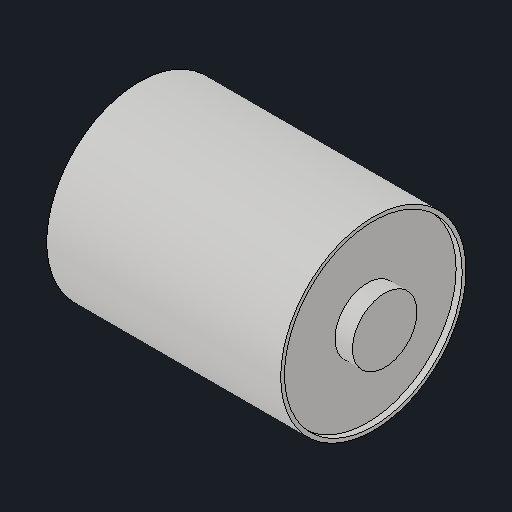
# Autodesk Inventor part: Silnik
Saved by Autodesk Inventor 2023 (Build 270158000, 158)
## iProperties
Created: 2022-01-30
Part Number: Silnik
Material: Ogólny
Document SubType Name: Modeling
Designer: Michał
Density: 4.22271 g/cm^3
Appearance: Domyślna
Mass: 60 g
Surface Area: 34.9646 cm^2
Volume: 14.2089 cm^3
Author: Michał
Autodesk Inventor part; units mm, degrees
ref_plane "YZ Plane" through (0, 0, 0) normal (1, 0, 0) x (0, 1, 0)
ref_plane "XZ Plane" through (0, 0, 0) normal (0, 1, 0) x (-1, 0, 0)
ref_plane "XY Plane" through (0, 0, 0) normal (0, 0, 1) x (1, 0, 0)
sketch "Szkic1" plane through (0, 0, 0) normal (1, 0, 0) x (0, 1, 0)
  circle A0 centre (0, 0) radius 12.2
  dimension "d0" = 24.4
  constraints: 1 centre point, 1 coincident
  measures "d0" diameter of A0
extrude "Wyciągnięcie proste1" add sketch "Szkic1" along normal blind 30.8
sketch "Szkic2" plane through (30.8, 0, 0) normal (1, 0, 0) x (0, 0, -1)
  circle A0 centre (0, 0) radius 11.7
  dimension "d3" = 23.4
  constraints: 1 centre point, 1 coincident
  measures "d3" diameter of A0
extrude "Wyciągnięcie proste2" cut sketch "Szkic2" against normal blind 0.8
sketch "Szkic3" plane through (30, 0, 0) normal (1, 0, 0) x (0, 0, -1)
  circle A0 centre (0, 0) radius 4.2479
  constraints: 1 centre point, 1 coincident
extrude "Wyciągnięcie proste3" add sketch "Szkic3" along normal blind 2.3
sketch "Szkic4" plane through (0, 0, 0) normal (-1, 0, 0) x (0, 0, 1)
  line L0 (0, 0) -> (8.5, 0) construction
  line L1 (0, 0) -> (-8.5, 0) construction
  dimension "d8" = 8.5
  constraints: 4 end point, 2 coincident, 2 horizontal, 1 collinear, 1 horizontal alignment
  measures "d8" distance of L0.start L0.end
hole "Otwór1" at (0, 0, 8.5) at (0, 0, -8.5) direction (1, 0, 0) diameter 2.459 depth 3 tip angle 118 thread size "M3x0.5" class "6H" standard "ISO Metric profile"
sketch "Szkic5" plane through (0, 0, 0) normal (-1, 0, 0) x (0, 0, 1)
  circle A0 centre (0, 0) radius 3.2
  dimension "d16" = 6.4
  constraints: 1 centre point, 1 coincident
  measures "d16" diameter of A0
extrude "Wyciągnięcie proste4" add sketch "Szkic5" along normal blind 1.6
